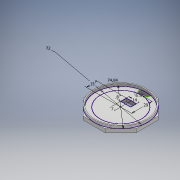
# Autodesk Inventor part: LEDR03
Saved by Autodesk Inventor 2018.1 (Build 221171000, 171)
## iProperties
Created: 2017-10-22
Part Number: LEDR03
Material: Generic
Document SubType Name: Modeling
Designer: s167968
Density: 1 g/cm^3
Appearance: Default
Author: s167968
Autodesk Inventor part; units mm, degrees
ref_plane "YZ Plane" through (0, 0, 0) normal (1, 0, 0) x (0, 1, 0)
ref_plane "XZ Plane" through (0, 0, 0) normal (0, 1, 0) x (-1, 0, 0)
ref_plane "XY Plane" through (0, 0, 0) normal (0, 0, 1) x (1, 0, 0)
sketch "Sketch1" plane through (0, 0, 0) normal (0, 0, 1) x (1, 0, 0)
  line L0 (37.4203, -15.5) -> (15.5, -37.4203)
  line L1 (15.5, -37.4203) -> (-15.5, -37.4203)
  line L2 (-15.5, -37.4203) -> (-37.4203, -15.5)
  line L3 (-37.4203, -15.5) -> (-37.4203, 15.5)
  line L4 (-37.4203, 15.5) -> (-15.5, 37.4203)
  line L5 (-15.5, 37.4203) -> (15.5, 37.4203)
  line L6 (15.5, 37.4203) -> (37.4203, 15.5)
  line L7 (37.4203, 15.5) -> (37.4203, -15.5)
  point P0 (0, 0)
  point P1 (0, 0)
  dimension "d0" = 31
  dimension "d1" = 0
  constraints: 16 end point, 1 coincident, 17 other
  measures "d0" distance of L4.end L5.end
  measures "d1" vertical distance of L4.end L5.end
extrude "Extrusion3" add sketch "Sketch1" along normal blind 5
sketch "Sketch5" plane through (0, 0, 5) normal (0, 0, 1) x (1, 0, 0)
  circle A0 centre (0, 0) radius 36
  circle A1 centre (0, 0) radius 37.42
  line L0 (-7, 15) -> (7, 15)
  line L1 (7, 15) -> (7, 7)
  line L2 (7, 7) -> (-7, 7)
  line L3 (-7, 7) -> (-7, 15)
  line L4 (0, 29) -> (0, 22) construction
  line L5 (0, 29) -> (7, 29) construction
  circle A2 centre (0, 0) radius 29
  line L6 (-6, 28.3725) -> (-7.9667, 35.1074)
  line L7 (6, 28.3725) -> (7.9667, 35.1074)
  dimension "d14" = 72
  dimension "d15" = 74.84
  dimension "d16" = 14
  dimension "d17" = 8
  dimension "d18" = 7
  dimension "d19" = 15
  dimension "d24" = 29
  dimension "d27" = 6
  dimension "d28" = 0
  constraints: 16 end point, 5 point on circle, 4 coincident, 3 centre point, 2 horizontal, 2 parallel, 2 perpendicular
  measures "d14" diameter of A0
  measures "d15" diameter of A1
  measures "d16" distance of L0.start L0.end
  measures "d17" distance of L2.end L0.start
  measures "d18" distance from line of point (0, 0) L3
  measures "d19" distance from line of L0 point (0, 0)
  measures "d24" distance of point (0, 29) point (0, 0)
  measures "d27" horizontal distance of L4.start L6.start
  measures "d28" horizontal distance of point (0, 0) L4.start
extrude "Extrusion4" add sketch "Sketch5" along normal blind 3.3 contours A1
extrude "Extrusion5" cut sketch "Sketch5" against normal blind 5 contours L0 L1 L2 L3
extrude "Extrusion6" cut sketch "Sketch5" against normal blind 5 contours L7 A2 L6 A0 picked at (-0.671, 33.577)
body "Solid1"
